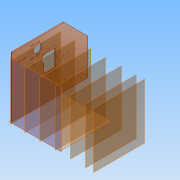
# Autodesk Inventor part: Pancake_LHS
Saved by Autodesk Inventor 2018.1 (Build 221171000, 171)
## iProperties
Created: 2019-02-21
Part Number: Pancake_LHS
Material: Wood (Oak)
Document SubType Name: Modeling
Designer: James
Density: 0.76 g/cm^3
Appearance: White Oak - Natural Medium Gloss
Author: James
Autodesk Inventor part; units mm, degrees
ref_plane "YZ Plane" through (0, 0, 0) normal (1, 0, 0) x (0, 1, 0)
ref_plane "XZ Plane" through (0, 0, 0) normal (0, 1, 0) x (-1, 0, 0)
ref_plane "XY Plane" through (0, 0, 0) normal (0, 0, 1) x (1, 0, 0)
derived "Pancake_Skeleton.ipt"
ref_plane "Ground" through (0, 0, 0) normal (0, 1, 0) x (-1, 0, 0)
ref_plane "Back" through (0, 0, 0) normal (0, 0, 1) x (1, 0, 0)
ref_plane "LHS" through (0, 0, 0) normal (1, 0, 0) x (0, 1, 0)
ref_plane "Lane 1" through (90, 0, 0) normal (1, 0, 0) x (0, 1, 0)
ref_plane "Lane 2" through (185, 0, 0) normal (1, 0, 0) x (0, 1, 0)
ref_plane "Lane 3" through (280, 0, 0) normal (1, 0, 0) x (0, 1, 0)
ref_plane "Lane 4" through (375, 0, 0) normal (1, 0, 0) x (0, 1, 0)
ref_plane "Lane 5" through (470, 0, 0) normal (1, 0, 0) x (0, 1, 0)
ref_plane "RHS" through (520, 0, 0) normal (1, 0, 0) x (0, 1, 0)
sketch "Sketch1" plane through (0, 0, 0) normal (1, 0, 0) x (0, 1, 0)
  line L0 (0, 450) -> (0, -75) projected
  line L1 (-95, 0) -> (570, 0) projected
  line L2 (0, 0) -> (475, 0)
  line L3 (475, 0) -> (475, 375)
  line L4 (475, 375) -> (0, 375)
  line L5 (0, 375) -> (0, 0)
  dimension "d1" = 475
  dimension "d2" = 375
  constraints: 8 end point, 2 parallel, 1 horizontal, 1 perpendicular
  measures "d1" distance of L4.end L3.end
  measures "d2" distance of L3.end L2.end
extrude "Extrusion1" add sketch "Sketch1" against normal blind 5
chamfer "Chamfer1" distance 150 angle 45 1 edges at (-2.5, 475, 375)
sketch "Sketch2" plane through (-5, 0, 0) normal (-1, 0, 0) x (0, 0, 1)
  line L0 (0, 0) -> (375, 0) projected
  line L1 (0, 570) -> (0, -95) projected
  point P0 (195, 355)
  point P1 (195, 320)
  dimension "d8" = 35
  dimension "d9" = 320
  dimension "d10" = 195
  constraints: 1 vertical alignment
  measures "d8" distance of point (195, 320) point (195, 355)
  measures "d9" distance from line of L0 point (195, 320)
  measures "d10" distance from line of point (195, 320) L1
hole "Hole1" at (-5, 355, 195) at (-5, 320, 195) direction (1, 0, 0) diameter 4.5 end through all clearance for "Socket Head Cap Screw" size "M4" standard "Ansi Metric M Profile"
sketch "Sketch3" plane through (-5, 0, 0) normal (-1, 0, 0) x (0, 0, 1)
  circle A0 centre (195, 320) radius 2.25 projected
  point P0 (0, 0)
  point P1 (148.666, 312)
  point P2 (65, 327)
  dimension "d18" = 130
  dimension "d19" = 7
  dimension "d20" = 85
  dimension "d21" = 15
  measures "d18" horizontal distance of A0.centre point (65, 327)
  measures "d19" vertical distance of A0.centre point (65, 327)
  measures "d20" distance of point (65, 327) point (148.666, 312)
  measures "d21" vertical distance of point (65, 327) point (148.666, 312)
hole "Hole2" at (-5, 312, 148.666) at (-5, 327, 65) direction (1, 0, 0) diameter 4.5 end through all clearance for "Socket Head Cap Screw" size "M4" standard "Ansi Metric M Profile"
sketch "Sketch4" plane through (-5, 0, 0) normal (-1, 0, 0) x (0, 0, 1)
  circle A0 centre (65, 327) radius 2.25 projected
  point P0 (0, 0)
  point P1 (20, 465)
  point P2 (20, 430)
  dimension "d29" = 35
  dimension "d30" = 103
  dimension "d31" = 45
  constraints: 1 vertical alignment
  measures "d29" distance of point (20, 430) point (20, 465)
  measures "d30" vertical distance of A0.centre point (20, 430)
  measures "d31" horizontal distance of A0.centre point (20, 430)
hole "Hole3" at (-5, 465, 20) at (-5, 430, 20) direction (1, 0, 0) diameter 4.5 end through all clearance for "Socket Head Cap Screw" size "M4" standard "Ansi Metric M Profile"
sketch "Sketch5" plane through (-5, 0, 0) normal (-1, 0, 0) x (0, 0, 1)
  line L0 (225, 475) -> (0, 475) projected
  line L1 (0, 570) -> (0, -95) projected
  circle A0 centre (20, 465) radius 2.25 projected
  point P0 (0, 0)
  point P1 (65, 457.5)
  dimension "d41" = 45
  dimension "d42" = 7.5
  measures "d41" horizontal distance of point (65, 457.5) A0.centre
  measures "d42" vertical distance of point (65, 457.5) A0.centre
hole "Hole4" at (-5, 457.5, 65) direction (1, 0, 0) diameter 3 end through all
sketch "Sketch6" plane through (-5, 0, 0) normal (-1, 0, 0) x (0, 0, 1)
  circle A0 centre (65, 457.5) radius 1.5 projected
  point P0 (0, 0)
  point P1 (65, 422.5)
  dimension "d50" = 35
  constraints: 1 vertical alignment
  measures "d50" distance of point (65, 422.5) A0.centre
hole "Hole5" [suppressed]
sketch "Sketch7" plane through (-5, 0, 0) normal (-1, 0, 0) x (0, 0, 1)
  circle A0 centre (65, 457.5) radius 1.5 projected
  point P0 (0, 0)
  point P1 (65, 433.5)
  point P2 (65, 411.5)
  dimension "d58" = 24
  dimension "d59" = 22
  constraints: 2 vertical alignment
  measures "d58" distance of point (65, 433.5) A0.centre
  measures "d59" distance of point (65, 411.5) point (65, 433.5)
hole "Hole6" at (-5, 433.5, 65) at (-5, 411.5, 65) direction (1, 0, 0) diameter 3.4 end through all clearance for "Socket Head Cap Screw" size "M3" standard "Ansi Metric M Profile"
sketch "Sketch9" plane through (-5, 0, 0) normal (-1, 0, 0) x (0, 0, 1)
  circle A0 centre (65, 327) radius 2.25 projected
  point P0 (0, 0)
  point P1 (119, 275)
  point P2 (119, 240)
  dimension "d67" = 35
  dimension "d68" = 54
  dimension "d69" = 52
  constraints: 1 vertical alignment
  measures "d67" distance of point (119, 240) point (119, 275)
  measures "d68" horizontal distance of point (119, 275) A0.centre
  measures "d69" vertical distance of point (119, 275) A0.centre
hole "Hole7" at (-5, 275, 119) at (-5, 240, 119) direction (1, 0, 0) diameter 4.5 end through all clearance for "Socket Head Cap Screw" size "M4" standard "Ansi Metric M Profile"
sketch "Sketch10" plane through (-5, 0, 0) normal (-1, 0, 0) x (0, 0, 1)
  circle A0 centre (119, 240) radius 2.25 projected
  point P0 (0, 0)
  point P1 (154, 143)
  point P2 (238.8528, 138)
  dimension "d77" = 85
  dimension "d81" = 97
  dimension "d190" = 5
  dimension "d192" = 35
  measures "d77" distance of point (238.853, 138) point (154, 143)
  measures "d81" vertical distance of A0.centre point (154, 143)
  measures "d190" vertical distance of point (238.853, 138) point (154, 143)
  measures "d192" horizontal distance of point (154, 143) A0.centre
hole "Hole8" at (-5, 143, 154) at (-5, 138, 238.8528) direction (1, 0, 0) diameter 4.5 end through all clearance for "Flat Head Machine Screw" size "M4" standard "Ansi Metric M Profile"
sketch "Sketch11" plane through (-5, 0, 0) normal (-1, 0, 0) x (0, 0, 1)
  line L0 (158, 270) -> (263, 270)
  line L1 (263, 270) -> (263, 200)
  line L2 (263, 200) -> (158, 200)
  line L3 (158, 200) -> (158, 270)
  line L4 (0, 0) -> (375, 0) projected
  line L5 (0, 570) -> (0, -95) projected
  circle A0 centre (119, 275) radius 2.25 projected
  dimension "d90" = 105
  dimension "d107" = 39
  dimension "d110" = 5
  dimension "d111" = 70
  constraints: 8 end point, 2 parallel, 1 horizontal, 1 perpendicular
  measures "d90" distance of L1.end L2.end
  measures "d107" distance from line of L3 A0.centre
  measures "d110" distance from line of A0.centre L0
  measures "d111" distance of L2.end L0.start
extrude "Extrusion2" cut sketch "Sketch11" against normal through all contours L0 L1 L2 L3
fillet "Fillet1" radius 5 4 edges at (-2.5, 270, 158) (-2.5, 200, 158) (-2.5, 200, 263) (-2.5, 270, 263)
sketch "Sketch12" plane through (-5, 0, 0) normal (-1, 0, 0) x (0, 0, 1)
  circle A0 centre (119, 275) radius 2.25 projected
  point P0 (0, 0)
  point P1 (142, 270)
  point P2 (142, 235)
  dimension "d97" = 35
  dimension "d98" = 23
  dimension "d99" = 5
  constraints: 1 vertical alignment
  measures "d97" distance of point (142, 235) point (142, 270)
  measures "d98" horizontal distance of A0.centre point (142, 270)
  measures "d99" vertical distance of point (142, 270) A0.centre
hole "Hole9" at (-5, 270, 142) at (-5, 235, 142) direction (1, 0, 0) diameter 4.5 end through all clearance for "Socket Head Cap Screw" size "M4" standard "Ansi Metric M Profile"
sketch "Sketch14" plane through (-5, 0, 0) normal (-1, 0, 0) x (0, 0, 1)
  line L0 (163, 270) -> (258, 270) projected
  line L1 (158, 205) -> (158, 265) projected
  circle A0 centre (142, 270) radius 2.25 projected
  point P0 (0, 0)
  point P1 (210.5, 278)
  point P2 (210.5, 193)
  dimension "d114" = 68.5
  dimension "d115" = 8
  dimension "d116" = 85
  constraints: 1 vertical alignment
  measures "d114" horizontal distance of point (210.5, 278) A0.centre
  measures "d115" vertical distance of A0.centre point (210.5, 278)
  measures "d116" distance of point (210.5, 193) point (210.5, 278)
hole "Hole10" at (-5, 278, 210.5) at (-5, 193, 210.5) direction (1, 0, 0) diameter 4.5 end through all clearance for "Socket Head Cap Screw" size "M4" standard "Ansi Metric M Profile"
sketch "Sketch15" plane through (-5, 0, 0) normal (-1, 0, 0) x (0, 0, 1)
  line L0 (263, 265) -> (263, 205) projected
  line L1 (163, 270) -> (258, 270) projected
  circle A0 centre (142, 270) radius 2.25 projected
  point P0 (0, 0)
  point P1 (279, 266)
  point P2 (279, 231)
  dimension "d126" = 137
  dimension "d127" = 4
  dimension "d157" = 35
  constraints: 1 vertical alignment
  measures "d126" horizontal distance of point (279, 266) A0.centre
  measures "d127" vertical distance of A0.centre point (279, 266)
  measures "d157" distance of point (279, 231) point (279, 266)
hole "Hole11" at (-5, 266, 279) at (-5, 231, 279) direction (1, 0, 0) diameter 4.5 end through all clearance for "Socket Head Cap Screw" size "M4" standard "Ansi Metric M Profile"
sketch "Sketch16" plane through (-5, 0, 0) normal (-1, 0, 0) x (0, 0, 1)
  line L0 (263, 265) -> (263, 205) projected
  line L1 (163, 270) -> (258, 270) projected
  point P0 (0, 0)
  point P1 (267, 192)
  point P2 (267, 162)
  dimension "d136" = 4
  dimension "d137" = 78
  dimension "d138" = 30
  constraints: 1 vertical alignment
  measures "d136" distance from line of point (267, 192) L0
  measures "d137" distance from line of point (267, 192) L1
  measures "d138" distance of point (267, 162) point (267, 192)
hole "Hole12" at (-5, 192, 267) at (-5, 162, 267) direction (1, 0, 0) diameter 4.5 end through all clearance for "Flat Head Machine Screw" size "M4" standard "Ansi Metric M Profile"
sketch "Sketch19" plane through (-5, 0, 0) normal (-1, 0, 0) x (0, 0, 1)
  circle A0 centre (279, 266) radius 2.25 projected
  circle A1 centre (142, 270) radius 2.25 projected
  line L0 (263, 265) -> (263, 205) projected
  line L1 (258, 200) -> (163, 200) projected
  point P0 (0, 0)
  point P1 (314, 160)
  point P2 (238, 210)
  dimension "d158" = 172
  dimension "d159" = 110
  dimension "d164" = 96
  dimension "d165" = 60
  measures "d158" horizontal distance of point (314, 160) A1.centre
  measures "d159" vertical distance of point (314, 160) A1.centre
  measures "d164" horizontal distance of point (238, 210) A1.centre
  measures "d165" vertical distance of A1.centre point (238, 210)
hole "Hole13" at (-5, 160, 314) at (-5, 210, 238) direction (1, 0, 0) diameter 50 end through all
sketch "Sketch20" plane through (-5, 0, 0) normal (-1, 0, 0) x (0, 0, 1)
  circle A0 centre (279, 231) radius 2.25 projected
  point P0 (0, 0)
  point P1 (279, 171)
  point P2 (279, 136)
  point P3 (349, 171)
  point P4 (349, 136)
  dimension "d166" = 60
  dimension "d167" = 35
  dimension "d168" = 70
  constraints: 3 vertical alignment, 2 horizontal alignment
  measures "d166" distance of point (279, 171) A0.centre
  measures "d167" distance of point (279, 136) point (279, 171)
  measures "d168" distance of point (349, 136) point (279, 136)
hole "Hole14" at (-5, 171, 279) at (-5, 136, 279) at (-5, 171, 349) at (-5, 136, 349) direction (1, 0, 0) diameter 4.5 end through all clearance for "Flat Head Machine Screw" size "M4" standard "Ansi Metric M Profile"
sketch "Sketch21" plane through (-5, 0, 0) normal (-1, 0, 0) x (0, 0, 1)
  circle A0 centre (279, 171) radius 2.25 projected
  point P0 (0, 0)
  point P1 (303.5, 89)
  point P2 (303.5, 54)
  dimension "d178" = 82
  dimension "d179" = 35
  dimension "d189" = 24.5
  constraints: 1 vertical alignment
  measures "d178" vertical distance of point (303.5, 89) A0.centre
  measures "d179" distance of point (303.5, 54) point (303.5, 89)
  measures "d189" horizontal distance of point (303.5, 89) A0.centre
hole "Hole15" at (-5, 89, 303.5) at (-5, 54, 303.5) direction (1, 0, 0) diameter 4.5 end through all clearance for "Flat Head Machine Screw" size "M4" standard "Ansi Metric M Profile"
sketch "Sketch23" plane through (-5, 0, 0) normal (-1, 0, 0) x (0, 0, 1)
  circle A0 centre (279, 171) radius 2.25 projected
  circle A1 centre (349, 171) radius 2.25 projected
  point P0 (0, 0)
  point P1 (314, 126)
  point P2 (314, 106)
  dimension "d193" = 20
  dimension "d194" = 35
  dimension "d195" = 35
  dimension "d196" = 45
  constraints: 1 vertical alignment
  measures "d193" distance of point (314, 106) point (314, 126)
  measures "d194" horizontal distance of point (314, 126) A0.centre
  measures "d195" horizontal distance of point (314, 126) A1.centre
  measures "d196" vertical distance of A0.centre point (314, 126)
hole "Hole16" at (-5, 126, 314) at (-5, 106, 314) direction (1, 0, 0) diameter 4.5 end through all clearance for "Flat Head Machine Screw" size "M4" standard "Ansi Metric M Profile"
sketch "Sketch24" plane through (-5, 0, 0) normal (-1, 0, 0) x (0, 0, 1)
  circle A0 centre (65, 411.5) radius 1.7 projected
  point P0 (0, 0)
  point P1 (70, 386.5)
  dimension "d204" = 25
  dimension "d205" = 5
  measures "d204" vertical distance of A0.centre point (70, 386.5)
  measures "d205" horizontal distance of A0.centre point (70, 386.5)
hole "Hole17" [suppressed]
sketch "Sketch25" plane through (-5, 0, 0) normal (-1, 0, 0) x (0, 0, 1)
  line L0 (279, 163) -> (279, 151) construction
  line L1 (276.75, 163) -> (276.75, 151)
  line L2 (281.25, 151) -> (281.25, 163)
  arc A0 (281.25, 163) -> (276.75, 163) centre (279, 163) ccw
  arc A1 (276.75, 151) -> (281.25, 151) centre (279, 151) ccw
  line L3 (349, 163) -> (349, 151) construction
  line L4 (346.75, 163) -> (346.75, 151)
  line L5 (351.25, 151) -> (351.25, 163)
  arc A2 (351.25, 163) -> (346.75, 163) centre (349, 163) ccw
  arc A3 (346.75, 151) -> (351.25, 151) centre (349, 151) ccw
  line L6 (349, 128) -> (349, 116) construction
  line L7 (346.75, 128) -> (346.75, 116)
  line L8 (351.25, 116) -> (351.25, 128)
  arc A4 (351.25, 128) -> (346.75, 128) centre (349, 128) ccw
  arc A5 (346.75, 116) -> (351.25, 116) centre (349, 116) ccw
  line L9 (279, 128) -> (279, 116) construction
  line L10 (276.75, 128) -> (276.75, 116)
  line L11 (281.25, 116) -> (281.25, 128)
  arc A6 (281.25, 128) -> (276.75, 128) centre (279, 128) ccw
  arc A7 (276.75, 116) -> (281.25, 116) centre (279, 116) ccw
  circle A8 centre (349, 171) radius 2.25 projected
  circle A9 centre (349, 136) radius 2.25 projected
  circle A10 centre (279, 136) radius 2.25 projected
  circle A11 centre (279, 171) radius 2.25 projected
  point P0 (0, 0)
  point P1 (279, 157)
  point P2 (349, 157)
  point P3 (349, 122)
  point P4 (279, 122)
  dimension "d213" = 2.25
  dimension "d214" = 2.25
  dimension "d215" = 2.25
  dimension "d216" = 2.25
  dimension "d217" = 12
  dimension "d218" = 12
  dimension "d219" = 35
  dimension "d220" = 20
  constraints: 32 end point, 16 point on circle, 16 tangent, 8 centre point, 6 horizontal alignment, 5 parallel, 4 midpoint, 4 vertical alignment, 2 point on line, 2 vertical
  measures "d213" radius of A0
  measures "d214" radius of A2
  measures "d215" radius of A6
  measures "d216" radius of A4
  measures "d217" distance of L0.start L0.end
  measures "d218" distance of L9.start L9.end
  measures "d219" distance of point (349, 122) point (349, 157)
  measures "d220" distance of A11.centre L0.end
extrude "Extrusion3" cut sketch "Sketch25" against normal through all contours A0 L2 A1 L1 | A2 L5 A3 L4 | A4 L8 A5 L7 | A6 L11 A7 L10
sketch "Sketch26" plane through (-5, 0, 0) normal (-1, 0, 0) x (0, 0, 1)
  line L0 (303.5, 81) -> (303.5, 69) construction
  line L1 (301.25, 81) -> (301.25, 69)
  line L2 (305.75, 69) -> (305.75, 81)
  arc A0 (305.75, 81) -> (301.25, 81) centre (303.5, 81) ccw
  arc A1 (301.25, 69) -> (305.75, 69) centre (303.5, 69) ccw
  line L3 (303.5, 46) -> (303.5, 34) construction
  line L4 (301.25, 46) -> (301.25, 34)
  line L5 (305.75, 34) -> (305.75, 46)
  arc A2 (305.75, 46) -> (301.25, 46) centre (303.5, 46) ccw
  arc A3 (301.25, 34) -> (305.75, 34) centre (303.5, 34) ccw
  circle A4 centre (303.5, 89) radius 2.25 projected
  point P0 (0, 0)
  point P1 (303.5, 75)
  point P2 (303.5, 40)
  dimension "d223" = 12
  dimension "d224" = 12
  dimension "d225" = 35
  dimension "d226" = 20
  dimension "d227" = 2.25
  dimension "d228" = 2.25
  constraints: 16 end point, 8 point on circle, 8 tangent, 4 centre point, 3 parallel, 2 midpoint, 2 vertical alignment, 1 vertical
  measures "d223" distance of L0.start L0.end
  measures "d224" distance of L3.start L3.end
  measures "d225" distance of point (303.5, 75) point (303.5, 40)
  measures "d226" distance of A4.centre L0.end
  measures "d227" radius of A0
  measures "d228" radius of A2
extrude "Extrusion4" cut sketch "Sketch26" against normal through all contours A0 L2 A1 L1 | A2 L5 A3 L4
equation "\"d194\" = d195"
equation "\"d214\" = d213"
equation "\"d215\" = d213"
equation "\"d216\" = d214"
equation "\"d218\" = d217"
equation "\"d224\" = d223"
equation "\"d228\" = d227"
body "Solid1"
